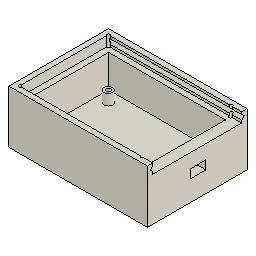
Crashsense Mark-1 Enclosure Part-1 v24 (Autodesk Fusion 360 design; units mm, degrees)
Autodesk Fusion 360 part; units mm, degrees
note: some values were not read from the file. Chosen so that the rebuilt part matches the saved one: which face or edge a step refers to. Set by a fixed rule: which sketch regions a step uses.
sketch "Sketch1" plane through (0, 0, 0) normal (0, 0, 1) x (1, 0, 0)
  line L0 (48.0125, -30.025) -> (-48.0125, -30.025)
  line L1 (-48.0125, -30.025) -> (-48.0125, 30.025)
  line L2 (-48.0125, 30.025) -> (48.0125, 30.025)
  line L3 (48.0125, 30.025) -> (48.0125, -30.025)
  line L4 (48.0125, -30.025) -> (-48.0125, 30.025) construction
  line L5 (-48.0125, -30.025) -> (48.0125, 30.025) construction
  line L6 (48.0125, 30.025) -> (43.9995, 30.025)
  line L7 (43.9995, 30.025) -> (43.9995, 25.755)
  circle A0 centre (43.9995, 25.755) radius 1.6
  line L8 (-48.0125, 30.025) -> (-43.9995, 30.025)
  line L9 (-43.9995, 30.025) -> (-43.9995, 25.755)
  circle A1 centre (-43.9995, 25.755) radius 1.6
  line L10 (48.0125, -30.025) -> (43.9995, -30.025)
  line L11 (43.9995, -30.025) -> (43.9995, -26.245)
  circle A2 centre (43.9995, -26.245) radius 1.6
  line L12 (-48.0125, -30.025) -> (-43.9995, -30.025)
  line L13 (-43.9995, -30.025) -> (-43.9995, -26.245)
  circle A3 centre (-43.9995, -26.245) radius 1.6
  line L14 (48.0125, -30.025) -> (-48.0125, -30.025)
  line L15 (-48.0125, -30.025) -> (-48.0125, 30.025)
  line L16 (-48.0125, 30.025) -> (48.0125, 30.025)
  line L17 (48.0125, 30.025) -> (48.0125, -30.025)
  line L18 (-54.0125, 36.025) -> (54.0125, 36.025)
  line L19 (54.0125, 36.025) -> (54.0125, -36.025)
  line L20 (54.0125, -36.025) -> (-54.0125, -36.025)
  line L21 (-54.0125, -36.025) -> (-54.0125, 36.025)
  line L22 (64.0125, -46.025) -> (-64.0125, -46.025)
  line L23 (-64.0125, -46.025) -> (-64.0125, 46.025)
  line L24 (-64.0125, 46.025) -> (64.0125, 46.025)
  line L25 (64.0125, 46.025) -> (64.0125, -46.025)
  dimension "d1" = 96.025
  dimension "d2" = 60.05
  dimension "d3" = 4.013
  dimension "d4" = 4.27
  dimension "d5" = 3.2
  dimension "d6" = 4.013
  dimension "d7" = 4.27
  dimension "d8" = 3.2
  dimension "d9" = 4.013
  dimension "d10" = 3.78
  dimension "d11" = 3.2
  dimension "d12" = 4.013
  dimension "d13" = 3.78
  dimension "d14" = 3.2
  dimension "d15" = 0
  dimension "d16" = -6
  dimension "d17" = -10
  constraint horizontal L0
  constraint perpendicular L0 L1
  constraint parallel L0 L2
  constraint parallel L1 L3
  constraint coincident L4 origin
  constraint coincident L5 origin
  constraint perpendicular L3 L6
  constraint perpendicular L6 L7
  constraint coincident L7.end A0.centre
  constraint perpendicular L1 L8
  constraint perpendicular L8 L9
  constraint coincident L9.end A1.centre
  constraint perpendicular L3 L10
  constraint perpendicular L0 L11
  constraint coincident L11.end A2.centre
  constraint perpendicular L1 L12
  constraint perpendicular L12 L13
  constraint coincident L13.end A3.centre
  measures "d1" distance of L1.end L2.end
  measures "d2" distance of L0.end L1.end
  measures "d3" distance of L2.end L6.end
  measures "d4" distance of L6.end L7.end
  measures "d5" diameter of A0
  measures "d6" distance of L1.end L8.end
  measures "d7" distance of L8.end L9.end
  measures "d8" diameter of A1
  measures "d9" distance of L0.start L10.end
  measures "d10" distance of L10.end L11.end
  measures "d11" diameter of A2
  measures "d12" distance of L0.end L12.end
  measures "d13" distance of L12.end L13.end
  measures "d14" diameter of A3
  measures "d15" distance of L3
extrude "Extrude1" add sketch "Sketch1" along normal blind 30 contours L22 L23 L24 L25 makes body 1
extrude "Extrude2" add sketch "Sketch1" against normal blind 10 separate body contours L0 L1 L2 L3 L6 L8 L10 L12 L14 L15 L16 L17 | L18 L19 L20 L21 makes body 2
extrude "Extrude3" add sketch "Sketch1" against normal blind 10 contours L22 L23 L24 L25 bodies 1 2
sketch "Sketch2" plane through (0, 0, 0) normal (0, 0, 1) x (-1, 0, 0)
  circle A0 centre (-43.9995, 26.245) radius 1.6
  circle A1 centre (-43.9995, -25.755) radius 1.6
  circle A2 centre (43.9995, 26.245) radius 1.6
  circle A3 centre (43.9995, -25.755) radius 1.6
  line L0 (54.0125, 36.025) -> (-54.0125, 36.025)
  line L1 (-54.0125, 36.025) -> (-54.0125, -36.025)
  line L2 (-54.0125, -36.025) -> (54.0125, -36.025)
  line L3 (54.0125, -36.025) -> (54.0125, 36.025)
  circle A4 centre (43.9995, -25.755) radius 4
  circle A5 centre (-43.9995, -25.755) radius 4
  circle A6 centre (43.9995, 26.245) radius 4
  circle A7 centre (-43.9995, 26.245) radius 4
  circle A8 centre (43.9995, -25.755) radius 1.6
  circle A9 centre (43.9995, -25.755) radius 2
  circle A10 centre (-43.9995, -25.755) radius 1.6
  circle A11 centre (-43.9995, -25.755) radius 2
  circle A12 centre (43.9995, 26.245) radius 1.6
  circle A13 centre (43.9995, 26.245) radius 2
  circle A14 centre (-43.9995, 26.245) radius 1.6
  circle A15 centre (-43.9995, 26.245) radius 2
  dimension "d24" = 8
  dimension "d25" = 8
  dimension "d26" = 8
  dimension "d27" = 8
  dimension "d28" = 3.2
  dimension "d29" = 4
  dimension "d30" = 3.2
  dimension "d31" = 4
  dimension "d32" = 3.2
  dimension "d33" = 4
  dimension "d34" = 3.2
  dimension "d35" = 4
  constraint concentric A3 A4
  constraint concentric A1 A5
  constraint concentric A2 A6
  constraint concentric A0 A7
  constraint concentric A3 A8
  constraint concentric A8 A9
  constraint concentric A5 A10
  constraint concentric A10 A11
  constraint concentric A6 A12
  constraint concentric A6 A13
  constraint concentric A7 A14
  constraint concentric A7 A15
  measures "d24" diameter of A4
  measures "d25" diameter of A5
  measures "d26" diameter of A6
  measures "d27" diameter of A7
  measures "d28" diameter of A8
  measures "d29" diameter of A9
  measures "d30" diameter of A10
  measures "d31" diameter of A11
  measures "d32" diameter of A12
  measures "d33" diameter of A13
  measures "d34" diameter of A14
  measures "d35" diameter of A15
delete_face "DeleteFace1" 1 faces at (44.1984, -24.6574, -6.6667) on bodies 1
delete_face "DeleteFace2" 1 faces at (-42.4075, -26.0857, -3.3333) on bodies 1
delete_face "DeleteFace3" 1 faces at (-42.4015, 25.6752, -6.6667) on bodies 1
delete_face "DeleteFace4" 1 faces at (44.1984, 27.3426, -6.6667) on bodies 1
extrude "Extrude4" add sketch "Sketch2" along normal blind 10 contours A0 A14 | A1 A10 | A2 A12 | A3 A8 | A4 | A5 | A6 | A7 | A9 | A11 | A13 | A15 bodies 1
sketch "Sketch4" plane through (0, 0, 10) normal (0, 0, 1) x (-1, 0, 0)
  circle A0 centre (43.9995, -25.755) radius 4
  circle A1 centre (43.9995, -25.755) radius 2
  dimension "d39" = 4
  constraint concentric A0 A1
  measures "d39" diameter of A1
extrude "Extrude5" cut sketch "Sketch4" against normal blind 3 contours A1 bodies 1
sketch "Sketch5" plane through (0, 0, 10) normal (0, 0, 1) x (-1, 0, 0)
  circle A0 centre (-43.9995, -25.755) radius 4
  circle A1 centre (-43.9995, -25.755) radius 2
  dimension "d42" = 4
  constraint concentric A0 A1
  measures "d42" diameter of A1
extrude "Extrude6" cut sketch "Sketch5" against normal blind 3 contours A1 bodies 1
sketch "Sketch6" plane through (0, 0, 10) normal (0, 0, 1) x (-1, 0, 0)
  circle A0 centre (-43.9995, 26.245) radius 4
  circle A1 centre (-43.9995, 26.245) radius 2
  dimension "d45" = 4
  constraint concentric A0 A1
  measures "d45" diameter of A1
extrude "Extrude7" cut sketch "Sketch6" against normal blind 3 contours A1 bodies 1
sketch "Sketch7" plane through (0, 0, 10) normal (0, 0, 1) x (-1, 0, 0)
  circle A0 centre (43.9995, 26.245) radius 4
  circle A1 centre (43.9995, 26.245) radius 2
  dimension "d48" = 4
  constraint concentric A0 A1
  measures "d48" diameter of A1
extrude "Extrude8" cut sketch "Sketch7" against normal blind 3 contours A1 bodies 1
extrude "Extrude9" cut 4 faces at (-44.1478, 25.105, 7) (-45.1474, -26.7978, 7) (42.8516, 25.2022, 7) (45.1474, -26.7978, 7) along direction (0, 0, -1) blind 2 on bodies 1 bodies 1
extrude "Extrude10" cut 4 faces at (45.1474, -26.7978, 5) (42.8516, 25.2022, 5) (-44.1478, 25.105, 5) (-45.1474, -26.7978, 5) along direction (0, 0, -1) blind 0.95 on bodies 1 bodies 1
sketch "Sketch8" plane through (64.0125, 0, 0) normal (1, 0, 0) x (0, 1, 0)
  line L0 (46.025, -10) -> (46.025, 30)
  line L1 (46.025, 30) -> (-46.025, 30)
  line L2 (-46.025, 30) -> (-46.025, -10)
  line L3 (-46.025, -10) -> (46.025, -10)
  line L4 (-46.025, 13) -> (0.975, 13)
  line L5 (0.975, 13) -> (0.975, -10)
  line L6 (8.975, 8) -> (-7.025, 8)
  line L7 (-7.025, 8) -> (-7.025, 18)
  line L8 (-7.025, 18) -> (8.975, 18)
  line L9 (8.975, 18) -> (8.975, 8)
  line L10 (8.975, 8) -> (-7.025, 18) construction
  line L11 (-7.025, 8) -> (8.975, 18) construction
  point P0 (0.975, 13)
  dimension "d55" = 47
  dimension "d56" = 23
  dimension "d57" = 16
  dimension "d58" = 10
  constraint coincident L2 L4.start
  constraint perpendicular L2 L4
  constraint perpendicular L4 L5
  constraint horizontal L6
  constraint perpendicular L6 L7
  constraint parallel L6 L8
  constraint parallel L7 L9
  constraint coincident L10 P0
  constraint coincident L11 P0
  constraint coincident P0 L4.end
  measures "d55" distance of L4.start P0
  measures "d56" distance of P0 L5.end
  measures "d57" distance of L7.end L8.end
  measures "d58" distance of L6.end L7.end
extrude "Extrude11" cut sketch "Sketch8" against normal blind 10 contours L4 L5 L6 L7 | L4 L5 L6 L7 L8 L9 bodies 1
extrude "Extrude12" add 1 faces at (60.6792, 8.975, 14.6667) along direction (0, -1, 0) blind 1 on bodies 1 bodies 1
extrude "Extrude13" add 1 faces at (60.6792, -7.025, 11.3333) along direction (0, 1, 0) blind 1 on bodies 1 bodies 1
extrude "Extrude14" add 1 faces at (60.6792, 3.3083, 8) along direction (0, 0, 1) blind 1 on bodies 1 bodies 1
extrude "Extrude15" add 1 faces at (60.6792, -1.3583, 18) along direction (0, 0, -1) blind 1 on bodies 1 bodies 1
sketch "Sketch9" plane through (0, 0, 30) normal (0, 0, 1) x (-1, 0, 0)
  line L0 (-54.0125, 36.025) -> (54.0125, 36.025)
  line L1 (54.0125, 36.025) -> (54.0125, -36.025)
  line L2 (54.0125, -36.025) -> (-54.0125, -36.025)
  line L3 (-54.0125, -36.025) -> (-54.0125, 36.025)
  line L4 (-64.0125, -46.025) -> (64.0125, -46.025)
  line L5 (64.0125, -46.025) -> (64.0125, 46.025)
  line L6 (64.0125, 46.025) -> (-64.0125, 46.025)
  line L7 (-64.0125, 46.025) -> (-64.0125, -46.025)
  line L8 (-54.0125, -36.025) -> (-54.0125, -46.025)
  line L9 (-54.0125, 36.025) -> (-54.0125, 46.025)
  line L10 (-54.0125, -41.025) -> (64.0125, -41.025)
  line L11 (-54.0125, 41.025) -> (64.0125, 41.025)
  line L12 (54.0125, -36.025) -> (64.0125, -36.025)
  line L13 (54.0125, 36.025) -> (64.0125, 36.025)
  line L14 (54.0125, 0) -> (64.0125, 0)
  line L15 (59.0125, -41.025) -> (59.0125, 41.025)
  line L16 (-54.0125, 41.025) -> (-64.0125, 41.025)
  line L17 (-54.0125, -41.025) -> (-64.0125, -41.025)
  line L18 (-54.0125, -46.025) -> (-64.0125, -46.025)
  line L19 (-64.0125, -41.025) -> (-64.0125, -46.025)
  line L20 (-64.0125, 41.025) -> (-64.0125, 46.025)
  line L21 (-54.0125, 46.025) -> (-64.0125, 46.025)
  point P0 (59.0125, 0)
  constraint coincident L2.end L3.start
  constraint coincident L4 L8.end
  constraint perpendicular L4 L8
  constraint coincident L0.start L3.end
  constraint coincident L6 L9.end
  constraint perpendicular L6 L9
  constraint midpoint L8 L10.start
  constraint coincident L5 L10.end
  constraint perpendicular L5 L10
  constraint midpoint L9 L11.start
  constraint coincident L5 L11.end
  constraint perpendicular L5 L11
  constraint coincident L1.end L2.start
  constraint coincident L5 L12.end
  constraint perpendicular L5 L12
  constraint coincident L0.end L1.start
  constraint coincident L5 L13.end
  constraint perpendicular L5 L13
  constraint midpoint L1 L14.start
  constraint midpoint L5 L14.end
  constraint midpoint L15 P0
  constraint coincident L14 P0
  constraint coincident L11 L15.end
  constraint perpendicular L11 L15
  constraint coincident L7 L16.end
  constraint perpendicular L7 L16
  constraint coincident L7 L17.end
  constraint perpendicular L7 L17
  constraint coincident L4.start L7.end
  constraint coincident L6.end L7.start
extrude "Extrude16" add sketch "Sketch9" along normal blind 4 contours L6 L7 L9 L16 L20 L21 | L5 L6 L9 L11 | L5 L11 L13 L15 | L5 L13 L14 L15 | L4 L5 L8 L10 | L4 L7 L8 L17 L18 L19 | L5 L12 L14 L15 | L5 L10 L12 L15 bodies 1
extrude "Extrude17" cut 1 faces at (-59.0125, 13.675, 32.6667) along direction (-1, 0, 0) blind 0.3 on bodies 1 bodies 1
sketch "Sketch10" plane through (0, 0, 34) normal (0, 0, 1) x (-1, 0, 0)
  line L0 (-64.0125, 41.025) -> (59.3125, 41.025)
  line L1 (59.3125, 41.025) -> (59.3125, -41.025)
  line L2 (59.3125, -41.025) -> (-64.0125, -41.025)
  line L3 (-64.0125, -41.025) -> (-64.0125, -46.025)
  line L4 (-64.0125, -46.025) -> (64.0125, -46.025)
  line L5 (64.0125, -46.025) -> (64.0125, 46.025)
  line L6 (64.0125, 46.025) -> (-64.0125, 46.025)
  line L7 (-64.0125, 46.025) -> (-64.0125, 41.025)
  line L8 (-54, 36) -> (-54, 41.025)
  line L9 (-54, -36) -> (-54, -41)
  circle A0 centre (-54, -41) radius 1.5
  line L10 (59.3125, -41.025) -> (59.3125, -40.725)
  line L11 (59.3125, 41.025) -> (58.7125, 41.025)
  line L12 (58.7125, 41.025) -> (58.7125, 40.425)
  circle A1 centre (58.7125, 40.425) radius 1.5
  line L13 (-54, 41.025) -> (-54, 40.725)
  circle A2 centre (-54, 40.725) radius 1.5
  line L14 (-54, -41) -> (-53.7, -41)
  line L15 (59.3125, -41.025) -> (58.7125, -41.025)
  line L16 (59.3125, -40.725) -> (58.7125, -40.725)
  circle A3 centre (58.7125, -40.725) radius 1.5
  dimension "d75" = 3
  dimension "d80" = 0.3
  dimension "d82" = 0.6
  dimension "d83" = 0.6
  dimension "d84" = 3
  dimension "d86" = 0.3
  dimension "d87" = 3
  dimension "d88" = 0.3
  dimension "d102" = 0.6
  dimension "d103" = 0.6
  dimension "d104" = 3
  constraint coincident L0 L8.end
  constraint perpendicular L0 L8
  constraint vertical L9
  constraint coincident L9.end A0.centre
  constraint perpendicular L2 L10
  constraint coincident L0.end L1.start
  constraint perpendicular L1 L11
  constraint perpendicular L11 L12
  constraint coincident L12.end A1.centre
  constraint coincident L13.end A2.centre
  constraint perpendicular L9 L14
  constraint coincident L1.end L2.start
  constraint perpendicular L1 L15
  constraint perpendicular L1 L16
  constraint coincident L16.end A3.centre
  measures "d75" diameter of A0
  measures "d80" distance of L1.end L10.end
  measures "d82" distance of L0.end L11.end
  measures "d83" distance of L11.end L12.end
  measures "d84" diameter of A1
  measures "d86" distance of L8.end L13.end
  measures "d87" diameter of A2
  measures "d88" distance of L9.end L14.end
  measures "d102" distance of L1.end L15.end
  measures "d103" distance of L10.end L16.end
  measures "d104" diameter of A3
extrude "Extrude25" cut sketch "Sketch10" against normal blind 20 contours L1 L2 L10 L15 A3 | L1 L2 L10 L15 A3 bodies 1
extrude "Extrude26" cut sketch "Sketch10" against normal blind 20 contours L0 L1 L11 A1 | L0 L1 L11 A1 bodies 1
extrude "Extrude27" cut sketch "Sketch10" against normal blind 20 contours L0 L1 L11 A1 | L0 L1 L11 A1 bodies 1
extrude "Extrude28" cut sketch "Sketch10" against normal blind 20 contours L0 L8 L13 A2 | L0 A2 | L0 L8 L13 A2 bodies 1
extrude "Extrude29" cut sketch "Sketch10" against normal blind 20 contours L2 A0 | L2 A0 bodies 1
extrude "Extrude30" add 1 faces at (-23.0084, -43.1778, 34) along direction (0, 0, 1) blind 5 on bodies 1 bodies 1
sketch "Sketch12" plane through (64.0125, 0, 0) normal (1, 0, 0) x (0, 1, 0)
  line L0 (7.975, 17) -> (7.975, 9)
  line L1 (7.975, 9) -> (-6.025, 9)
  line L2 (-6.025, 9) -> (-6.025, 17)
  line L3 (-6.025, 17) -> (7.975, 17)
  line L4 (46.025, -10) -> (46.025, 39)
  line L5 (46.025, 39) -> (41.025, 39)
  line L6 (41.025, 39) -> (41.025, 30)
  line L7 (41.025, 30) -> (-41.025, 30)
  line L8 (-41.025, 30) -> (-41.025, 39)
  line L9 (-41.025, 39) -> (-46.025, 39)
  line L10 (-46.025, 39) -> (-46.025, -10)
  line L11 (-46.025, -10) -> (46.025, -10)
  line L12 (-41.025, 30) -> (-41.025, 39)
  line L13 (-46.025, 39) -> (-46.025, 30)
  line L14 (-41.025, 39) -> (-46.025, 39)
  line L15 (-46.025, 30.0835) -> (-41.025, 30)
  line L16 (-41.025, 34.5) -> (-46.025, 34.5)
  line L17 (-41.025, 39) -> (-41.025, 34.5)
  line L18 (-41.025, 30) -> (-41.025, 34.5)
  line L19 (-41.025, 36.75) -> (-43.525, 34.5)
  line L20 (-41.025, 32.25) -> (-43.525, 34.5)
  line L21 (0, 40) -> (0, -10)
  line L22 (-41.025, 36.75) -> (-41.025, 32.25)
  line L23 (41.025, 36.75) -> (43.525, 34.5)
  line L24 (41.025, 32.25) -> (43.525, 34.5)
  line L25 (41.025, 30) -> (41.025, 39)
  dimension "d119" = 4.5
  dimension "d120" = 9
  constraint coincident L7.end L8.start
  constraint coincident L8.end L9.start
  constraint coincident L9.end L10.start
  constraint coincident L10 L13.end
  constraint coincident L10 L15.start
  constraint midpoint L12 L16.start
  constraint perpendicular L8 L16
  constraint midpoint L17 L19.start
  constraint midpoint L16 L19.end
  constraint midpoint L18 L20.start
  constraint midpoint L11 L21.end
  constraint perpendicular L11 L21
  constraint symmetric L7.end L21 L6.end
  constraint symmetric L8.end L21 L5.end
  constraint symmetric L19.start L21 L23.start
  constraint symmetric L19.end L21 L23.end
  constraint symmetric L20.start L21 L24.start
  measures "d119" distance of L16.start L7.end
  measures "d120" distance of L9.end L13.end
extrude "Extrude31" cut sketch "Sketch12" against normal blind 123.325 contours L6 L23 L24 L25 | L8 L12 L16 L18 L20 L22 | L8 L12 L16 L17 L19 L22 bodies 1
extrude "Extrude18" [suppressed]
sketch "Sketch11" plane through (0, 0, 34) normal (0, 0, 1) x (-1, 0, 0)
  line L0 (59.3125, -41.025) -> (57.5428, -41.025)
  line L1 (59.3125, -39.2553) -> (59.3125, -41.025)
  arc A0 (57.5428, -41.025) -> (59.3125, -39.2553) centre (59.0125, -40.725) ccw
extrude "Extrude19" [suppressed]
extrude "Extrude20" [suppressed]
extrude "Extrude21" [suppressed]
extrude "Extrude22" [suppressed]
extrude "Extrude23" [suppressed]
delete_face "DeleteFace5" [suppressed]
extrude "Extrude24" [suppressed]
